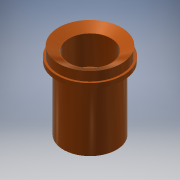
# Autodesk Inventor part: Phenolic 8-inch v1
Saved by Autodesk Inventor 2017 (Build 210142000, 142)
## iProperties
Created: 2016-01-09
Part Number: Phenolic 8-inch v1
Material: Phenolic Resin
Document SubType Name: Modeling
Designer: Jared
Density: 1.38 g/cm^3
Appearance: Smooth - Light Orange
Author: Jared
Autodesk Inventor part; units mm, degrees
ref_plane "YZ Plane" through (0, 0, 0) normal (1, 0, 0) x (0, 1, 0)
ref_plane "XZ Plane" through (0, 0, 0) normal (0, 1, 0) x (-1, 0, 0)
ref_plane "XY Plane" through (0, 0, 0) normal (0, 0, 1) x (1, 0, 0)
sketch "Sketch1" plane through (0, 0, 0) normal (0, 0, 1) x (1, 0, 0)
  line L0 (-87.8501, 55.3459) -> (-87.8501, 29.9459)
  line L1 (-87.8501, 29.9459) -> (-93.4, 29.9459)
  line L2 (-59.2667, 42.6459) -> (-60.6149, 42.6459)
  line L3 (-59.2667, 42.6459) -> (0, 42.6459) construction
  line L4 (-41.4694, -37.9453) -> (-35.1194, -37.9453)
  line L5 (-93.4, 29.9459) -> (-93.4, 17.2459)
  line L6 (-93.4, 17.2459) -> (-80.7, 17.2459)
  line L7 (-80.7, 17.2459) -> (-74.35, 17.2459)
  line L8 (-74.35, 17.2459) -> (-74.35, -160.6575)
  line L9 (-93.4, 17.2459) -> (-93.4, 7.7209)
  line L10 (-93.4, 17.2459) -> (-83.875, 17.2459) construction
  line L11 (-93.4, 7.7209) -> (-80.7, 7.7209)
  line L12 (-80.7, 7.7209) -> (-80.7, -43.0791)
  line L13 (-80.7, -43.0791) -> (-93.4, -43.0791)
  line L14 (-93.4, 7.7209) -> (-87.05, 7.7209)
  line L15 (-87.05, 7.7209) -> (-87.05, 1.7773)
  line L16 (-87.05, 1.7773) -> (-93.4, 1.7773)
  line L17 (-93.4, 29.9459) -> (-93.4, 7.7209)
  line L18 (-93.4, 1.7773) -> (-93.4, -43.0791)
  line L19 (-80.7, -43.0791) -> (-21.9625, -43.0791) construction
  line L20 (-68, -160.6575) -> (-74.35, -160.6575)
  line L21 (-64.6621, -148.2003) -> (-40.1276, -148.2003) construction
  line L22 (0, 42.6459) -> (0, 0)
  line L23 (-87.8501, 55.3459) -> (-18.3062, 55.3459) construction
  line L24 (-87.8501, 55.3459) -> (-14.7047, 55.3459) construction
  line L25 (-87.8501, 55.3459) -> (-55.5582, 40.2879)
  line L26 (-87.8501, 55.3459) -> (-52.22, 55.3459) construction
  line L27 (-59.2667, 42.6459) -> (-59.2667, -37.9453)
  line L28 (-59.2667, 42.6459) -> (21.3245, 42.6459) construction
  line L29 (-59.2667, -37.9453) -> (-41.4694, -37.9453)
  line L30 (-74.35, -160.6575) -> (-35.1194, -37.9453)
  dimension "d87" = 25.4
  dimension "d88" = 5.5499
  dimension "d89" = 87.8501
  dimension "d90" = 12.7
  dimension "d92" = 59.2667
  dimension "d93" = 6.35
  dimension "d95" = 12.7
  dimension "d96" = 12.7
  dimension "d97" = 6.35
  dimension "d98" = 9.525
  dimension "d99" = 50.8
  dimension "d100" = 12.7
  dimension "d101" = 6.35
  dimension "d102" = 5.9436
  dimension "d113" = 25
  dimension "d115" = 32.2919
  dimension "d117" = 80.5912
  constraints: 63 end point, 12 horizontal, 11 perpendicular, 3 equal length, 3 point on line, 3 vertical, 2 collinear, 1 midpoint, 1 parallel, 1 vertical alignment, 1 other
  measures "d87" distance of L0.start L0.end
  measures "d88" distance of L0.end L5.start
  measures "d89" distance from line of L22.end L0
  measures "d90" vertical distance of L2.start L0.start
  measures "d92" horizontal distance of L22.end L2.start
  measures "d93" distance of L4.start L4.end
  measures "d95" distance of L5.start L5.end
  measures "d96" distance of L5.end L7.start
  measures "d97" distance of L7.start L8.start
  measures "d98" distance of L5.end L17.end
  measures "d99" distance of L11.end L19.start
  measures "d100" distance of L17.end L11.end
  measures "d101" distance of L17.end L14.end
  measures "d102" distance of L14.end L16.start
  measures "d113" angle of L25 L26
  measures "d115" horizontal distance of L0.start L25.end
  measures "d117" distance of L2.start L29.start
revolve "Revolution2" add sketch "Sketch1" angle 360 about axis through (0, 42.6459, 0) along (0, -1, 0) contours L25 L27 L29 L4 L30 L8 L7 L6 L5 L1 L0 | L2 L27 L25
body "Solid2"
